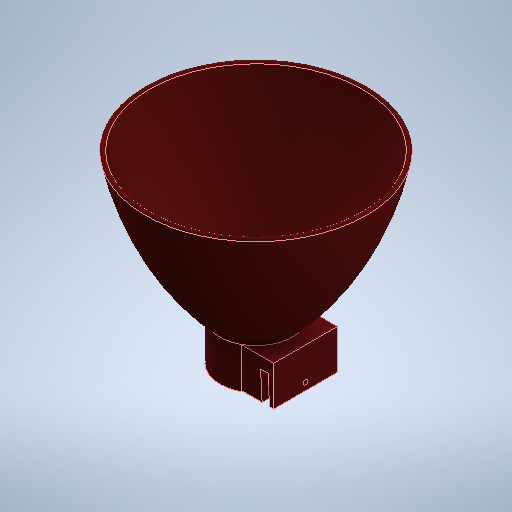
# Autodesk Inventor part: Cone FV
Saved by Autodesk Inventor 2025.4 (Build 294407000, 407)
## iProperties
Created: 2026-04-10
Part Number: Cone FV
Material: Generic
Document SubType Name: Modeling
Designer: lenovo
Density: 1 g/cm^3
Appearance: Default(1)
Author: lenovo
Autodesk Inventor part; units mm, degrees
ref_plane "XZ Plane" through (0, 0, 0) normal (0, 1, 0) x (-1, 0, 0)
ref_plane "XY Plane" through (0, 0, 0) normal (0, 0, 1) x (1, 0, 0)
sketch "Sketch1" plane through (0, 0, 0) normal (0, 0, 1) x (1, 0, 0)
  line L0 (0, 0) -> (0, 130)
  line L1 (22.5, 0) -> (22.5, 30)
  arc A0 (22.5, 30) -> (75, 130) centre (-121.124, 169.1839) ccw
  arc A1 (25.5, 28.7901) -> (77.9419, 129.4122) centre (-121.124, 169.1839) ccw
  line L2 (25.5, 28.7901) -> (25.5, 0)
  arc A2 (77.9419, 129.4122) -> (75, 130) centre (76.4709, 129.7061) ccw
  line L3 (22.5, 0) -> (25.5, 0)
  dimension "d0" = 30
  dimension "d1" = 200
  dimension "d2" = 100
  dimension "d3" = 45
  dimension "d4" = 150
  dimension "d5" = 3
  constraints: 8 end point, 6 point on circle, 3 centre point, 2 horizontal alignment, 2 tangent, 2 vertical, 1 horizontal, 1 other
  measures "d0" distance of L1.start L1.end
  measures "d1" radius of A0
  measures "d2" vertical distance of L1.end A0.end
  measures "d3" diameter of L1 L0
  measures "d4" diameter of A0.end L0
  measures "d5" radial gap between concentric circles of A0 A1
revolve "Revolution1" add sketch "Sketch1" angle 360 about axis through (0, 0, 0) along (0, 1, 0)
ref_plane "Work Plane1" through (35, 0, 0) normal (1, 0, 0) x (0, 1, 0)
sketch "Sketch2" plane through (35, 0, 0) normal (1, 0, 0) x (0, 1, 0)
  line L0 (0.7901, 22.5) -> (28.7901, 22.5)
  line L1 (28.7901, 22.5) -> (28.7901, -22.5)
  line L2 (28.7901, -22.5) -> (0.7901, -22.5)
  line L3 (0.7901, -22.5) -> (0.7901, 22.5)
  line L4 (0.7901, 22.5) -> (28.7901, -22.5) construction
  line L5 (28.7901, 22.5) -> (0.7901, -22.5) construction
  line L6 (28.7901, -25.5) -> (28.7901, 25.5) projected
  point P0 (0, 0)
  point P1 (14.7901, 0)
  point P2 (28.7901, 0)
  point P3 (28.7901, 0)
  dimension "d16" = 0
  dimension "d8" = 45
  dimension "d9" = 28
  constraints: 12 end point, 4 midpoint, 2 parallel, 1 coincident, 1 horizontal, 1 perpendicular, 1 point on line
  measures "d8" distance of L2.end L0.start
  measures "d9" distance of L1.end L2.end
extrude "Extrusion1" add sketch "Sketch2" against normal up to next
sketch "Sketch3" plane through (35, 0.7901, 22.5) normal (0, 0, 1) x (1, 0, 0)
  line L0 (-4.0467, 19.9726) -> (-3, 0)
  line L1 (-3, 0) -> (-8.1929, -0.2721)
  line L2 (-8.1929, -0.2721) -> (-9.2396, 19.7004)
  line L3 (-9.2396, 19.7004) -> (-4.0467, 19.9726)
  line L4 (-4.0467, 19.9726) -> (-8.1929, -0.2721) construction
  line L5 (-3, 0) -> (-9.2396, 19.7004) construction
  line L6 (0, 28) -> (0, 0) projected
  line L7 (0, 0) -> (-23, 0) projected
  point P0 (-35, -0.7901)
  point P1 (-6.1198, 9.8502)
  point P2 (-6.1198, 9.8502)
  point P3 (0, 14)
  point P4 (-8.2071, 0)
  dimension "d12" = 93
  dimension "d13" = 5.2
  dimension "d14" = 20
  dimension "d15" = 3
  constraints: 12 end point, 4 midpoint, 2 parallel, 1 perpendicular, 1 point on line
  measures "d12" angle of L0 L7
  measures "d13" distance of L0.end L1.end
  measures "d14" distance of L0.start L0.end
  measures "d15" distance of L6.end L0.end
extrude "Extrusion2" cut sketch "Sketch3" against normal through all contours L0 L7 L2 L3
sketch "Sketch4" plane through (25.7604, 20.4906, 22.5) normal (0.9986, 0.0523, 0) x (0, 0, -1)
  circle A0 centre (22.5, -15) radius 1.65
  line L0 (45, -19.7275) -> (0, -19.7275) projected
  line L1 (0, 0) -> (45, 0) projected
  point P0 (22.5, -19.1143)
  point P1 (22.5, -19.7275)
  dimension "d18" = 3.3
  dimension "d19" = 15
  constraints: 1 centre point, 1 midpoint, 1 vertical alignment
  measures "d18" diameter of A0
  measures "d19" distance from line of A0.centre L1
extrude "Extrusion3" cut sketch "Sketch4" along normal mid plane 25
body "Solid1"
